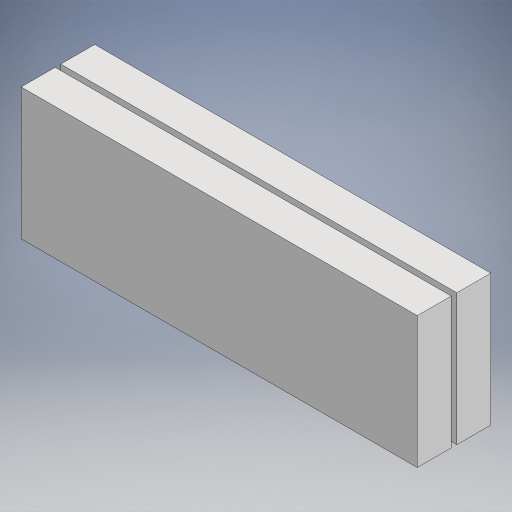
# Autodesk Inventor part: Part2
Saved by Autodesk Inventor 2023.2 (Build 272271000, 271)
## iProperties
Created: 2023-01-01
Part Number: Part2
Material: Generic
Document SubType Name: Modeling
Designer: awelt
Mass: 40004.9 g
Surface Area: 14109.6 cm^2
Volume: 40004.9 cm^3
Density: 1 g/cm^3
Appearance: Default
RuleStatus: InUse
BeforeDocSave0: file://C:\Users\awelt\Documents\Inventor\iLogic_Rules\BoundingStore
DocClose0: file://C:\Users\awelt\Documents\Inventor\iLogic_Rules\BoundingStore
Author: awelt
BoundingBL1: 6 1/2
BoundingBL2: 11 5/8
BoundingBL3: 35
BoundingCF: 1.53
Autodesk Inventor part; units mm, degrees
ref_plane "YZ Plane" through (0, 0, 0) normal (1, 0, 0) x (0, 1, 0)
ref_plane "XZ Plane" through (0, 0, 0) normal (0, 1, 0) x (-1, 0, 0)
ref_plane "XY Plane" through (0, 0, 0) normal (0, 0, 1) x (1, 0, 0)
sketch "Sketch2" plane through (0, 0, 0) normal (1, 0, 0) x (0, 1, 0)
  line L0 (0, 0) -> (295.275, 0)
  line L1 (295.275, 0) -> (295.275, -165.1)
  line L2 (295.275, -165.1) -> (0, -165.1)
  line L3 (0, -165.1) -> (0, 0)
  line L4 (295.275, -82.55) -> (0, -82.55) construction
  line L5 (295.275, -76.2) -> (0, -76.2)
  line L6 (0, -88.9) -> (295.275, -88.9)
  dimension "d3" = 295.275
  dimension "d4" = 165.1
  dimension "d5" = 12.7
  constraints: 14 end point, 4 point on line, 3 perpendicular, 2 midpoint, 2 parallel, 1 horizontal, 1 other
  measures "d3" distance of L1.end L2.end
  measures "d4" distance of L0.end L1.end
  measures "d5" distance of L6.end L5.start
extrude "Extrusion1" add sketch "Sketch2" along normal blind 889 contours L0 L1 L5 L3 | L6 L1 L2 L3
body "Solid1"
